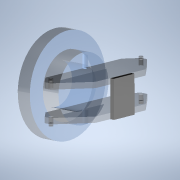
# Autodesk Inventor part: Part7
Saved by Autodesk Inventor 2022 (Build 260153000, 153)
## iProperties
Created: 2023-12-01
Part Number: Part7
Material: Generic
Document SubType Name: Modeling
Designer: harshidd
Density: 1 g/cm^3
Appearance: Red
Author: harshidd
Autodesk Inventor part; units mm, degrees
ref_plane "YZ Plane" through (0, 0, 0) normal (1, 0, 0) x (0, 1, 0)
ref_plane "XY Plane" through (0, 0, 0) normal (0, 0, 1) x (1, 0, 0)
sketch "Sketch1" plane through (0, 0, 0) normal (0, 0, 1) x (1, 0, 0)
  circle A0 centre (0, 0) radius 35
  dimension "d0" = 70
  constraints: 1 centre point, 1 coincident
  measures "d0" diameter of A0
extrude "Extrusion1" add sketch "Sketch1" along normal blind 10
sketch "Sketch2" plane through (0, 0, 10) normal (0, 0, 1) x (1, 0, 0)
  circle A0 centre (0, 0) radius 23
  dimension "d3" = 46
  constraints: 1 centre point, 1 coincident
  measures "d3" diameter of A0
extrude "Extrusion2" add sketch "Sketch2" along normal blind 13
ref_plane "Work Plane1" through (0, 13, 0) normal (0, 1, 0) x (-1, 0, 0)
sketch "Sketch3" plane through (0, 13, 0) normal (0, 1, 0) x (-1, 0, 0)
  line L0 (23, 23) -> (-23, 23) construction
  line L1 (0, 23) -> (57.0465, 23) construction
  line L2 (0, 23) -> (35, 23)
  line L3 (35, 23) -> (44.4682, 30.9448)
  line L4 (44.4682, 30.9448) -> (44.4682, 35.9448)
  line L5 (44.4682, 35.9448) -> (44.4682, 57.7443) construction
  line L6 (23, 23) -> (23, 67.0504) construction
  line L7 (0, 23) -> (0, 90.4674) construction
  line L8 (44.4682, 35.9448) -> (23, 53.9588)
  line L9 (0, 53.9588) -> (23, 53.9588)
  line L10 (0, 23) -> (-35, 23)
  line L11 (-35, 23) -> (-44.4682, 30.9448)
  line L12 (-44.4682, 30.9448) -> (-44.4682, 35.9448)
  line L13 (-44.4682, 35.9448) -> (-44.4682, 57.7443) construction
  line L14 (-44.4682, 35.9448) -> (-23, 53.9588)
  line L15 (0, 53.9588) -> (-23, 53.9588)
  point P0 (0, 0)
  dimension "d7" = 35
  dimension "d8" = 5
  dimension "d9" = 40
  dimension "d10" = 50
  constraints: 30 end point, 5 symmetric about line, 4 vertical, 3 point on line, 1 horizontal, 1 midpoint, 1 perpendicular
  measures "d7" distance of L1.start L2.end
  measures "d8" distance of L3.end L4.end
  measures "d9" angle of L1 L3
  measures "d10" angle of L5 L8
extrude "Extrusion3" add sketch "Sketch3" against normal blind 4
fillet "Fillet1" radius 2 6 edges at (-44.4682, 11, 30.9448) (-44.4682, 11, 35.9448) (-23, 11, 53.9588) (23, 11, 53.9588) (44.4682, 11, 35.9448) (44.4682, 11, 30.9448)
sketch "Sketch4" plane through (0, 13, 0) normal (0, 1, 0) x (1, 0, 0)
  line L0 (-44.4682, -31.8774) -> (-44.4682, -35.0122) construction
  line L1 (-44.4682, -33.4448) -> (-41.4682, -33.4448) construction
  circle A0 centre (-41.4682, -33.4448) radius 1.5
  point P0 (0, 0)
  dimension "d14" = 3
  dimension "d15" = 3
  constraints: 2 end point, 1 centre point, 1 coincident, 1 horizontal, 1 midpoint
  measures "d14" distance of L1.start L1.end
  measures "d15" diameter of A0
extrude "Extrusion4" cut sketch "Sketch4" against normal blind 4
sketch "Sketch5" plane through (0, 13, 0) normal (0, 1, 0) x (1, 0, 0)
  circle A0 centre (-41.4682, -33.4448) radius 1.5 projected
  circle A1 centre (-41.4682, -33.4448) radius 1.5
  point P0 (0, 0)
  constraints: 1 centre point, 1 coincident
extrude "Extrusion5" add sketch "Sketch5" along normal blind 2
sketch "Sketch6" plane through (-41.4682, 15, 33.4448) normal (0, 1, 0) x (1, 0, 0)
  circle A0 centre (0, 0) radius 1.5 projected
  circle A1 centre (0, 0) radius 1
  point P0 (41.4682, 33.4448)
  dimension "d20" = 0.5
  constraints: 1 centre point
  measures "d20" radial gap between concentric circles of A0 A1
extrude "Extrusion6" cut sketch "Sketch6" against normal blind 0.5 contours A1
mirror "Mirror1" about plane through (0, 0, 0) normal (1, 0, 0) of "Extrusion6", "Extrusion5", "Extrusion4"
mirror "Mirror2" about plane through (0, 0, 0) normal (0, 1, 0) of "Extrusion3", "Extrusion5", "Extrusion6", "Extrusion4", "Mirror1", "Fillet1"
sketch "Sketch7" plane through (0, 0, 23) normal (0, 0, 1) x (1, 0, 0)
  line L0 (-22.2721, 13) -> (22.2721, 13) projected
  line L1 (0, 13) -> (1, 13)
  line L2 (1, 13) -> (-1, 13)
  line L3 (-1, 13) -> (-1, 22)
  line L4 (-1, 22) -> (1, 22)
  line L5 (1, 22) -> (1, 13)
  point P0 (0, 0)
  dimension "d23" = 1
  dimension "d24" = 2
  dimension "d25" = 9
  dimension "d26" = 2
  constraints: 10 end point, 2 perpendicular, 2 point on line, 1 midpoint
  measures "d23" distance of L1.start L1.end
  measures "d24" distance of L1.end L2.end
  measures "d25" distance of L2.end L3.end
  measures "d26" distance of L3.end L4.end
extrude "Extrusion7" add sketch "Sketch7" along normal blind 3
fillet "Fillet2" radius 1 2 edges at (1, 22, 24.5) (-1, 22, 24.5)
mirror "Mirror3" about plane through (0, 0, 0) normal (0, 1, 0) of "Fillet2", "Extrusion7"
sketch "Sketch9" plane through (-22.2721, 13, 53.9588) normal (0, 0, 1) x (1, 0, 0)
  line L0 (31.7721, -26) -> (12.7721, -26)
  line L1 (12.7721, -26) -> (12.7721, 0)
  line L2 (12.7721, 0) -> (31.7721, 0)
  line L3 (31.7721, 0) -> (31.7721, -26)
  line L4 (31.7721, -26) -> (12.7721, 0) construction
  line L5 (12.7721, -26) -> (31.7721, 0) construction
  point P0 (22.2721, -13)
  dimension "d30" = 19
  dimension "d31" = 26
  constraints: 12 end point, 2 midpoint, 2 parallel, 1 horizontal, 1 perpendicular
  measures "d30" distance of L1.end L2.end
  measures "d31" distance of L0.end L1.end
extrude "Extrusion8" add sketch "Sketch9" along normal blind 3 separate body
sketch "Sketch10" plane through (0, 0, 0) normal (0, 0, -1) x (-1, 0, 0)
  circle A0 centre (0, 0) radius 15
  dimension "d34" = 30
  constraints: 1 centre point, 1 coincident
  measures "d34" diameter of A0
extrude "Extrusion9" cut sketch "Sketch10" against normal blind 20 bodies 1
body "Solid1"
body "Solid2"
